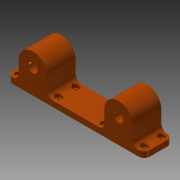
# Autodesk Inventor part: z arm wall bracket
Saved by Autodesk Inventor 2013 (Build 170138000, 138)
## iProperties
Created: 2013-07-22
Part Number: z arm wall bracket
Material: Generic
Document SubType Name: Modeling
Designer: employee
Density: 1 g/cm^3
Mass: 44.4062 g
Surface Area: 136.469 cm^2
Volume: 44.4062 cm^3
Author: employee
Autodesk Inventor part; units mm, degrees
ref_plane "YZ Plane" through (0, 0, 0) normal (1, 0, 0) x (0, 1, 0)
ref_plane "XZ Plane" through (0, 0, 0) normal (0, 1, 0) x (-1, 0, 0)
ref_plane "XY Plane" through (0, 0, 0) normal (0, 0, 1) x (1, 0, 0)
sketch "Sketch1" plane through (0, 0, 0) normal (0, 1, 0) x (-1, 0, 0)
  line L0 (-50, 0) -> (-50, 21)
  arc A0 (-25, 21) -> (-50, 21) centre (-37.5, 21) ccw
  line L1 (-25, 21) -> (-25, 5)
  line L2 (-25, 5) -> (25, 5)
  line L3 (25, 5) -> (25, 21)
  arc A1 (50, 21) -> (25, 21) centre (37.5, 21) ccw
  line L4 (50, 21) -> (50, 0)
  line L5 (50, 0) -> (-50, 0)
  circle A2 centre (-37.5, 21) radius 4.05
  circle A3 centre (37.5, 21) radius 4.05
  line L6 (-50, 5) -> (-60, 5)
  line L7 (-60, 5) -> (-60, 0)
  line L8 (-60, 0) -> (-50, 0)
  line L9 (50, 0) -> (60, 0)
  line L10 (60, 0) -> (60, 5)
  line L11 (60, 5) -> (50, 5)
  point P0 (0, 0)
  point P1 (0, 0)
  point P2 (0, 5)
  dimension "d0" = 5
  dimension "d2" = 21
  dimension "d3" = 12.5
  dimension "d4" = 8.1
  dimension "d5" = 75
  dimension "d8" = 10
  constraints: 24 end point, 6 parallel, 4 centre point, 4 perpendicular, 4 point on circle, 4 tangent, 3 coincident, 3 collinear, 2 equal length, 2 midpoint, 2 point on line, 1 equal radius, 1 vertical, 1 vertical alignment
  measures "d0" distance between parallel lines of L2 L5
  measures "d2" distance of L0.start L0.end
  measures "d3" radius of A0
  measures "d4" diameter of A3
  measures "d5" distance between parallel lines of L3 L0
  measures "d8" distance of L4.end L9.end
extrude "Extrusion1" add sketch "Sketch1" along normal blind 25
sketch "Sketch2" plane through (60, 0, 0) normal (0, 0, -1) x (-1, 0, 0)
  line L0 (0, 0) -> (120, 0) projected
  line L1 (0, 25) -> (120, 25) projected
  line L2 (0, 0) -> (0, 25) projected
  line L3 (10, 0) -> (35, 0) projected
  line L4 (10, 0) -> (10, 25) projected
  line L5 (35, 25) -> (10, 25) projected
  line L6 (35, 0) -> (35, 25) projected
  line L7 (85, 0) -> (110, 0) projected
  line L8 (85, 0) -> (85, 25) projected
  line L9 (110, 25) -> (85, 25) projected
  line L10 (110, 0) -> (110, 25) projected
  line L11 (5, 20) -> (40, 20)
  line L12 (40, 20) -> (40, 5)
  line L13 (40, 5) -> (5, 5)
  line L14 (5, 5) -> (5, 20)
  line L15 (80, 20) -> (115, 20)
  line L16 (115, 20) -> (115, 5)
  line L17 (115, 5) -> (80, 5)
  line L18 (80, 5) -> (80, 20)
  circle A0 centre (5, 20) radius 1.55
  circle A1 centre (5, 5) radius 1.55
  circle A2 centre (40, 5) radius 1.55
  circle A3 centre (40, 20) radius 1.55
  circle A4 centre (80, 20) radius 1.55
  circle A5 centre (80, 5) radius 1.55
  circle A6 centre (115, 5) radius 1.55
  circle A7 centre (115, 20) radius 1.55
  point P0 (60, 0)
  point P1 (22.5, 20)
  point P2 (22.5, 25)
  point P3 (97.5, 20)
  point P4 (97.5, 25)
  point P5 (5, 12.5)
  point P6 (10, 12.5)
  point P7 (80, 12.5)
  point P8 (85, 12.5)
  dimension "d9" = 5
  dimension "d10" = 5
  dimension "d11" = 3.1
  constraints: 16 end point, 8 centre point, 8 coincident, 8 midpoint, 7 equal radius, 4 parallel, 2 equal length, 2 horizontal, 2 horizontal alignment, 2 perpendicular, 2 vertical alignment
  measures "d9" distance between parallel lines of L2 L14
  measures "d10" distance between parallel lines of L1 L11
  measures "d11" diameter of A7
extrude "Extrusion2" cut sketch "Sketch2" against normal blind 2.5 contours A1 L14 L13 | L13 L14 A1 | A2 L12 L13 | L13 L12 A2 | A0 L14 L11 | L11 L14 A0 | A5 L18 L17 | L17 L18 A5 | A3 L12 L11 | L11 L12 A3 | A6 L16 L17 | L17 L16 A6 | A4 L18 L15 | L15 L18 A4 | A7 L16 L15 | L15 L16 A7
sketch "Sketch3" plane through (-20, 20, 2.5) normal (0, 0, -1) x (-1, 0, 0)
  circle A0 centre (35, 0) radius 1.55 projected
  circle A1 centre (0, -15) radius 1.55 projected
  circle A2 centre (-40, 0) radius 1.55 projected
  circle A3 centre (-75, -15) radius 1.55 projected
  circle A4 centre (-75, 0) radius 1.55 projected
  circle A5 centre (-40, -15) radius 1.55 projected
  circle A6 centre (0, 0) radius 1.55 projected
  circle A7 centre (35, -15) radius 1.55 projected
  line L0 (40, 5) -> (40, -20) projected
  line L1 (40, -20) -> (-80, -20) projected
  line L2 (-80, -20) -> (-80, 5) projected
  line L3 (-80, 5) -> (40, 5) projected
  line L4 (-71.7668, 0) -> (-73.3834, -2.8)
  line L5 (-73.3834, -2.8) -> (-76.6166, -2.8)
  line L6 (-76.6166, -2.8) -> (-78.2332, 0)
  line L7 (-78.2332, 0) -> (-76.6166, 2.8)
  line L8 (-76.6166, 2.8) -> (-73.3834, 2.8)
  line L9 (-73.3834, 2.8) -> (-71.7668, 0)
  line L10 (-71.7668, -15) -> (-73.3834, -17.8)
  line L11 (-73.3834, -17.8) -> (-76.6166, -17.8)
  line L12 (-76.6166, -17.8) -> (-78.2332, -15)
  line L13 (-78.2332, -15) -> (-76.6166, -12.2)
  line L14 (-76.6166, -12.2) -> (-73.3834, -12.2)
  line L15 (-73.3834, -12.2) -> (-71.7668, -15)
  line L16 (-43.2332, -15) -> (-41.6166, -12.2)
  line L17 (-41.6166, -12.2) -> (-38.3834, -12.2)
  line L18 (-38.3834, -12.2) -> (-36.7668, -15)
  line L19 (-36.7668, -15) -> (-38.3834, -17.8)
  line L20 (-38.3834, -17.8) -> (-41.6166, -17.8)
  line L21 (-41.6166, -17.8) -> (-43.2332, -15)
  line L22 (-43.2332, 0) -> (-41.6166, 2.8)
  line L23 (-41.6166, 2.8) -> (-38.3834, 2.8)
  line L24 (-38.3834, 2.8) -> (-36.7668, 0)
  line L25 (-36.7668, 0) -> (-38.3834, -2.8)
  line L26 (-38.3834, -2.8) -> (-41.6166, -2.8)
  line L27 (-41.6166, -2.8) -> (-43.2332, 0)
  line L28 (-3.2332, 0) -> (-1.6166, 2.8)
  line L29 (-1.6166, 2.8) -> (1.6166, 2.8)
  line L30 (1.6166, 2.8) -> (3.2332, 0)
  line L31 (3.2332, 0) -> (1.6166, -2.8)
  line L32 (1.6166, -2.8) -> (-1.6166, -2.8)
  line L33 (-1.6166, -2.8) -> (-3.2332, 0)
  line L34 (-3.2332, -15) -> (-1.6166, -12.2)
  line L35 (-1.6166, -12.2) -> (1.6166, -12.2)
  line L36 (1.6166, -12.2) -> (3.2332, -15)
  line L37 (3.2332, -15) -> (1.6166, -17.8)
  line L38 (1.6166, -17.8) -> (-1.6166, -17.8)
  line L39 (-1.6166, -17.8) -> (-3.2332, -15)
  line L40 (31.7668, -15) -> (33.3834, -12.2)
  line L41 (33.3834, -12.2) -> (36.6166, -12.2)
  line L42 (36.6166, -12.2) -> (38.2332, -15)
  line L43 (38.2332, -15) -> (36.6166, -17.8)
  line L44 (36.6166, -17.8) -> (33.3834, -17.8)
  line L45 (33.3834, -17.8) -> (31.7668, -15)
  line L46 (31.7668, 0) -> (33.3834, 2.8)
  line L47 (33.3834, 2.8) -> (36.6166, 2.8)
  line L48 (36.6166, 2.8) -> (38.2332, 0)
  line L49 (38.2332, 0) -> (36.6166, -2.8)
  line L50 (36.6166, -2.8) -> (33.3834, -2.8)
  line L51 (33.3834, -2.8) -> (31.7668, 0)
  point P0 (-20, -20)
  dimension "d14" = 5.6
  constraints: 96 end point, 8 coincident, 7 equal length, 7 horizontal, 1 horizontal alignment, 104 other
  measures "d14" distance between parallel lines of L8 L5
extrude "Extrusion3" cut sketch "Sketch3" against normal through all contours A0 | A1 | A2 | A3 | A4 | A5 | A6 | A7 | L4 L5 L6 L7 L8 L9 | L10 L11 L12 L13 L14 L15 | L16 L17 L18 L19 L20 L21 | L22 L23 L24 L25 L26 L27 | L28 L29 L30 L31 L32 L33 | L34 L35 L36 L37 L38 L39 | L40 L41 L42 L43 L44 L45 | L46 L47 L48 L49 L50 L51
fillet "Fillet1" radius 5 4 edges at (25, 12.5, 5) (50, 12.5, 5) (-25, 12.5, 5) (-50, 12.5, 5)
fillet "Fillet2" radius 5 4 edges at (-60, 25, 2.5) (-60, 0, 2.5) (60, 25, 2.5) (60, 0, 2.5)
body "Solid1"
